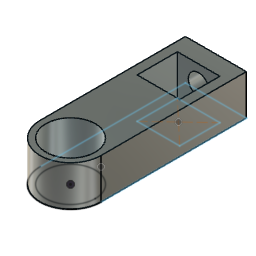
Pen Fixture - Bottom v5 (Autodesk Fusion 360 design; units mm, degrees)
Autodesk Fusion 360 part; units mm, degrees
sketch "Sketch1" plane through (0, 0, 0) normal (0, 0, 1) x (1, 0, 0)
  circle A0 centre (0, 0) radius 5.461
  line L0 (-6.731, 0) -> (-6.731, 32.131)
  line L1 (6.731, 0) -> (6.731, 32.131)
  line L2 (4.699, 19.431) -> (-4.699, 19.431)
  line L3 (-4.699, 19.431) -> (-4.699, 28.321)
  line L4 (-4.699, 28.321) -> (4.699, 28.321)
  line L5 (4.699, 28.321) -> (4.699, 19.431)
  line L6 (4.699, 19.431) -> (-4.699, 28.321) construction
  line L7 (-4.699, 19.431) -> (4.699, 28.321) construction
  line L8 (-6.731, 32.131) -> (6.731, 32.131)
  arc A1 (-6.731, 0) -> (6.731, 0) centre (0, 0) ccw
  point P0 (0, 23.876)
  point P1 (0, 6.731)
  dimension "d1" = 10.922
  dimension "d2" = 13.462
  dimension "d5" = 9.398
  dimension "d6" = 8.89
  dimension "d7" = 12.7
  dimension "d8" = 3.81
  constraint coincident A0.centre A1.centre
  constraint tangent L1 A1
  constraint horizontal L2
  constraint perpendicular L2 L3
  constraint parallel L2 L4
  constraint parallel L3 L5
  constraint coincident L6 P0
  constraint coincident L7 P0
  constraint coincident P1 A1
  constraint coincident L0 L8.start
  constraint perpendicular L0 L8
  measures "d1" diameter of A0
  measures "d2" diameter of A1
  measures "d5" distance of L3.end L4.end
  measures "d6" distance of L2.end L3.end
  measures "d7" distance of L2 P1
  measures "d8" distance of L4 L8
extrude "Extrude1" add sketch "Sketch1" along normal blind 8.89
sketch "Sketch3" plane through (0, 32.131, 0) normal (0, 1, 0) x (-1, 0, 0)
  line L0 (-6.731, 0) -> (6.731, 0)
  line L1 (6.731, 0) -> (6.731, 8.89)
  line L2 (6.731, 8.89) -> (-6.731, 8.89)
  line L3 (-6.731, 8.89) -> (-6.731, 0)
  line L4 (0, 8.89) -> (0, 7.239)
  circle A0 centre (0, 4.953) radius 2.286
  dimension "d12" = 1.651
  dimension "d13" = 4.572
  constraint midpoint L2 L4.start
  constraint perpendicular L2 L4
  constraint coincident L4.end A0
  measures "d12" distance of L4.start L4.end
  measures "d13" diameter of A0
extrude "Extrude2" cut sketch "Sketch3" against normal blind 5.842 contours A0
sketch "Sketch4" plane through (0, 0, 8.89) normal (0, 0, 1) x (-1, 0, 0)
  circle A0 centre (0, 0) radius 5.461
  line L0 (4.699, -28.321) -> (-4.699, -28.321)
  line L1 (-4.699, -28.321) -> (-4.699, -19.431)
  line L2 (-4.699, -19.431) -> (4.699, -19.431)
  line L3 (4.699, -19.431) -> (4.699, -28.321)
  line L4 (6.731, -32.131) -> (6.731, 0)
  arc A1 (6.731, 0) -> (-6.731, 0) centre (0, 0) ccw
  line L5 (-6.731, 0) -> (-6.731, -32.131)
  line L6 (-6.731, -32.131) -> (6.731, -32.131)
sketch "Sketch5" plane through (0, 0, 0) normal (0, 0, 1) x (1, 0, 0)
  line L0 (-3.048, 20.6883) -> (3.048, 20.6883)
  line L1 (3.048, 20.6883) -> (3.048, 10.6044)
  line L2 (3.048, 10.6044) -> (-3.048, 10.6044)
  line L3 (-3.048, 10.6044) -> (-3.048, 20.6883)
  point P0 (0, 10.6044)
  dimension "d18" = 6.096
  constraint horizontal L0
  constraint vertical L1
  constraint horizontal L2
  constraint vertical L3
  constraint midpoint L2 P0
  constraint vertical P0 origin
  measures "d18" distance of L1.end L2.end
extrude "Extrude3" cut sketch "Sketch5" along normal blind 6.35
